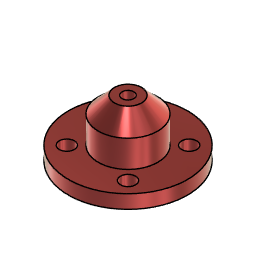
Flange 2mm v7 (Autodesk Fusion 360 design; units mm, degrees)
Autodesk Fusion 360 part; units mm, degrees
sketch "Sketch1" plane through (0, 0, 0) normal (0, 0, 1) x (1, 0, 0)
  circle A0 centre (0, 0) radius 11
  dimension "d1" = 22
  constraint coincident A0.centre origin
  measures "d1" diameter of A0
extrude "Extrude1" add sketch "Sketch1" along normal blind 2.5
sketch "Sketch2" plane through (0, 0, 2.5) normal (0, 0, 1) x (-1, 0, 0)
  circle A0 centre (0, 0) radius 11
  circle A1 centre (0, 0) radius 5.5
  dimension "d4" = 11
  constraint coincident A0.centre A1.centre
  measures "d4" diameter of A1
extrude "Extrude2" add sketch "Sketch2" along normal blind 8 contours A1
sketch "Sketch3" plane through (0, 0, 2.5) normal (0, 0, 1) x (-1, 0, 0)
  circle A0 centre (0, 0) radius 5.5
  circle A1 centre (0, 0) radius 11
  circle A2 centre (5.6569, -5.6569) radius 1.4
  circle A3 centre (5.6569, 5.6569) radius 1.4
  circle A4 centre (-5.6569, 5.6569) radius 1.4
  circle A5 centre (-5.6569, -5.6569) radius 1.4
  line L0 (0, 0) -> (7.7782, -7.7782) construction
  line L1 (0, 0) -> (11, 0) construction
  dimension "d7" = 2.8
  dimension "d8" = 8
  dimension "d10" = 360
  dimension "d27" = 45
  constraint horizontal L1
  constraint coincident A0.centre A1.centre
  constraint coincident A1 L0.end
  constraint coincident A2.centre L0
  constraint coincident A1 L1.end
  measures "d7" diameter of A2
  measures "d8" distance of A0.centre A2.centre
  measures "d27" angle of L0 L1
extrude "Extrude3" cut sketch "Sketch3" against normal through all contours A2 | A3 | A4 | A5
sketch "Sketch4" plane through (0, 0, 10.5) normal (0, 0, 1) x (-1, 0, 0)
  circle A0 centre (0, 0) radius 5.5
  circle A1 centre (0, 0) radius 1.1
  dimension "d12" = 2.2
  constraint coincident A0.centre A1.centre
  measures "d12" diameter of A1
extrude "Extrude4" cut sketch "Sketch4" against normal through all contours A1
chamfer "Chamfer1" distance 3 angle 45 1 edges at (5.1278, 1.9889, 10.5)
